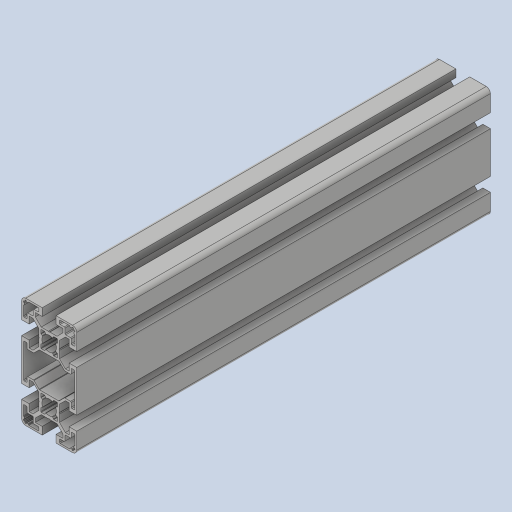
# Autodesk Inventor part: HFSLB8-4080-300
Saved by Autodesk Inventor 2023 (Build 270158000, 158)
## iProperties
Created: 2024-09-13
Part Number: HFSLB8-4080-300
Material: Generic
Catalog Web Link: www.cadenas.de
Description: NEFS8-4080, NEFSB8-4080, NEFSY8-4080, EFS8-4080, EFSB8-4080, HFS8-4080, HFSB8-4080, CAF8-4080, NFSL8-4080, HFSL8-4080, HFSLB8-4080, GFS8-4080, HFSY8-4080-Aluminum Frames -8 Series-2 Row Groove 40x80 mm Square-Specified Length
Vendor: MISUMI
Document SubType Name: Modeling
Designer: psAdmin
Manufacturer: MISUMI
Mass: 238.133 g
Surface Area: 2732.8 cm^2
Volume: 238.133 cm^3
Density: 1 g/cm^3
Appearance: PSOLRGB-175-175-175
Category: PARTsolutions
Company: MISUMI
PSOL_IDENT_0: {$CADENAS_DATA/23d-libs/misumi/metric/38_al_extrusions_blackets/8/hfs8_4080.prj},740 {VTYP=3D},{NB=H
PSOL_IDENT_1: FSLB8-4080-300},{LINA=HFSLB8-4080-300},{NN=NEFS8-4080, NEFSB8-4080, NEFSY8-4080, EFS8-4080, EFSB8-40
PSOL_IDENT_2: 80, HFS8-4080, HFSB8-4080, CAF8-4080, NFSL8-4080, HFSL8-4080, HFSLB8-4080, GFS8-4080, HFSY8-4080},{D
PSOL_IDENT_3: ATE=31.01.2024 10:05:59},{GEOMDATE=26.07.2023 02:49:00},{VERSION=},{LINEID=70},{WBVAR=L,ALT1,ALT2,AL
PSOL_IDENT_4: T4,ALT5,CP5,DL5,DR5,ALT6,ALT9,ALT10,ALT11,HP6,NHL6,DL6,NHR6,DR6,ALT7,ALT8,NH9,AH,BH,CH,DH,EH,NH10,AV
PSOL_IDENT_5: ,BV,CV,DV,EV,NH11,AP,BP,CP,DP,EP,ALT12,ALT13,Z,NH12,XA,XB,XC,XD,XE,NH13,YA,YB,YC,YD,YE,ALT14,HP14,DL
PSOL_IDENT_6: 14,DR14,ALT15,HP15,DL15,DR15,ALT16,HP16,DL16,DR16,ALT17,HQ17,JLP,ALT18,HQ18,KLP,ALT19,ALT20},{WBNUME
PSOL_IDENT_7: RIC=L,NH9,AH,BH,CH,DH,EH,NH10,AV,BV,CV,DV,EV,NH11,AP,BP,CP,DP,EP,NH12,XA,XB,XC,XD,XE,NH13,YA,YB,YC,Y
PSOL_IDENT_8: D,YE,HQ17,JLP,HQ18,KLP}  {NB=HFSLB8-4080-300},{LINA=HFSLB8-4080-300},{KT=DUMMY},{PN=HFSLB8-4080-300}
PSOL_IDENT_9: ,{TPS=HFSLB8-4080},{MAT=A6N01SS-T5 Aluminum Alloy},{ST=Black Anodize},{FRMW=40},{FRMH=80},{FRD=10.5}
PSOL_IDENT_10: ,{L=300},{MASS=2.12},{SA=785},{LX=13.4x10^4},{LY=52.9x10^4},{ALT1=},{M1=0},{IDM1=10.106},{DPL1=0},{D
PSOL_IDENT_11: PR1=0},{ALT1PN=},{ALT2=},{ALT2ALG= '','w/o End Tapping (Insert)','LHP','with LHP (Tapping on the Lef
PSOL_IDENT_12: t (Insert))','RHP','with RHP (Tapping on the Right (Insert))','HPW','with HPW (Tapping on Both Ends
PSOL_IDENT_13: (Insert))' },{M2=0},{DP2=0},{ALT2PN=},{ALT4=},{ALT4ALG= '', 'w/o SC (High Precision Cut)', 'SC', 'wi
PSOL_IDENT_14: th SC (High Precision Cut)' },{ALT4PN=},{ALT5=},{ALT5ALG= '','w/o 45 Degree Cut','1','with 45 Degree
PSOL_IDENT_15: Cut' },{CP5=},{CP5ALG= '','N/A' },{DL5=},{DL5ALG= '','N/A' },{DR5=},{DR5ALG= '','N/A' },{FRMLALT5=0
PSOL_IDENT_16: },{FRMRALT5=0},{ALT5PN=},{ALT6=},{ALT6ALG= '','w/o Fastening Location Wrench Access Hole Alterations'
PSOL_IDENT_17: ,'1','with Fastening Location Wrench Access Hole Alterations' },{ALT9=},{ALT9ALG= '','w/o Location S
PSOL_IDENT_18: pecified Wrench Access Hole Alteratons (Horizontal)','1','with Location Specified Wrench Access Hole
PSOL_IDENT_19: Alteratons (Horizontal)' },{ALT10=},{ALT10ALG= '','w/o Location Specified Wrench Access Hole Altera
PSOL_IDENT_20: tons (Vertical)','1','with Location Specified Wrench Access Hole Alteratons (Vertical)' },{ALT11=},{
PSOL_IDENT_21: ALT11ALG= '','w/o Location Specified Wrench Access Hole Alteratons (Crisscross)','1','with Location
PSOL_IDENT_22: Specified Wrench Access Hole Alteratons (Crisscross)' },{HP6=},{HP6ALG= '','N/A' },{NHL6=},{NHL6ALG=
PSOL_IDENT_23: '','N/A' },{DL6=},{DL6ALG= '','N/A' },{NHR6=},{NHR6ALG= '','N/A' },{DR6=},{DR6ALG= '','N/A' },{HL6=
PSOL_IDENT_24: 0},{HL6D=0},{HR6=0},{HR6D=0},{J6=0},{J6D=0},{K6=0},{K6D=0},{DD6=0},{DD6ALG=0},{ALT7=},{ALT7ALG= '','
PSOL_IDENT_25: N/A' },{ALT8=},{ALT8ALG= '','N/A' },{ALT678PN=},{NH9=0},{NH9MAX=5},{NH9ALG=[0]},{AH=0.0},{AHMIN=7},{
PSOL_IDENT_26: AHMAX=295},{AHALG=[0]},{BH=0.0},{BHMIN=2},{BHMAX=297},{BHALG=[0]},{CH=0.0},{CHMIN=2},{CHMAX=299},{CH
PSOL_IDENT_27: ALG=[0]},{DH=0.0},{DHMIN=2},{DHMAX=301},{DHALG=[0]},{EH=0.0},{EHMIN=2},{EHMAX=293},{EHALG=[0]},{NH10=
PSOL_IDENT_28: 0},{NH10MAX=5},{NH10ALG=[0]},{AV=0.0},{AVMIN=7},{AVMAX=295},{AVALG=[0]},{BV=0.0},{BVMIN=2},{BVMAX=29
PSOL_IDENT_29: 7},{BVALG=[0]},{CV=0.0},{CVMIN=2},{CVMAX=299},{CVALG=[0]},{DV=0.0},{DVMIN=2},{DVMAX=301},{DVALG=[0]}
PSOL_IDENT_30: ,{EV=0.0},{EVMIN=2},{EVMAX=293},{EVALG=[0]},{NH11=0},{NH11MAX=5},{NH11ALG=[0]},{AP=0.0},{APMIN=7},{A
PSOL_IDENT_31: PMAX=295},{APALG=[0]},{BP=0.0},{BPMIN=2},{BPMAX=297},{BPALG=[0]},{CP=0.0},{CPMIN=2},{CPMAX=299},{CPA
PSOL_IDENT_32: LG=[0]},{DP=0.0},{DPMIN=2},{DPMAX=301},{DPALG=[0]},{EP=0.0},{EPMIN=2},{EPMAX=293},{EPALG=[0]},{ALT9P
PSOL_IDENT_33: N=},{ALT10PN=},{ALT11PN=},{ALT91011PN=},{ALT12=},{ALT12ALG= '','w/o Counterbore Hole in Specified Po
PSOL_IDENT_34: sition (Vertical)','1','with Counterbore Hole in Specified Position (Vertical)' },{ALT13=},{ALT13ALG=
PSOL_IDENT_35: '','w/o Counterbore Hole in Specified Position (Horizontal)','1','with Counterbore Hole in Specifie
PSOL_IDENT_36: d Position (Horizontal)' },{Z=},{ZALG= '','N/A' },{DD12=0.0},{DD112=0.0},{NH12=0},{NH12MAX=5},{NH12A
PSOL_IDENT_37: LG=[0]},{XA=0.0},{XAMIN=7},{XAMAX=295},{XAALG=[0]},{XB=0.0},{XBMIN=2},{XBMAX=297},{XBALG=[0]},{XC=0.
PSOL_IDENT_38: 0},{XCMIN=2},{XCMAX=299},{XCALG=[0]},{XD=0.0},{XDMIN=2},{XDMAX=301},{XDALG=[0]},{XE=0.0},{XEMIN=2},{
PSOL_IDENT_39: XEMAX=293},{XEALG=[0]},{NH13=0},{NH13MAX=5},{NH13ALG=[0]},{YA=0.0},{YAMIN=7},{YAMAX=295},{YAALG=[0]}
PSOL_IDENT_40: ,{YB=0.0},{YBMIN=2},{YBMAX=297},{YBALG=[0]},{YC=0.0},{YCMIN=2},{YCMAX=299},{YCALG=[0]},{YD=0.0},{YDM
PSOL_IDENT_41: IN=2},{YDMAX=301},{YDALG=[0]},{YE=0.0},{YEMIN=2},{YEMAX=293},{YEALG=[0]},{ALT12PN=},{ALT13PN=},{ALT1
PSOL_IDENT_42: 213PN=},{ALT14=},{ALT14ALG= '','w/o D Type Hole Alteration','1','with D Type Hole Alteration' },{HP1
PSOL_IDENT_43: 4=},{HP14ALG= '','N/A' },{DL14=},{DL14ALG= '','N/A' },{DR14=},{DR14ALG= '','N/A' },{H14=0},{D14=0.0}
PSOL_IDENT_44: ,{ALT14PN=},{ALT15=},{ALT15ALG= '','w/o S Type Hole Alteration','1','with S Type Hole Alteration' },
PSOL_IDENT_45: {HP15=},{HP15ALG= '','N/A' },{DL15=},{DL15ALG= '','N/A' },{DR15=},{DR15ALG= '','N/A' },{H15=0},{D115=
PSOL_IDENT_46: 0.0},{D215=0.0},{ALT15PN=},{ALT16=},{ALT16ALG= '','w/o M Type Hole Alteration','1','with M Type Hole
PSOL_IDENT_47: Alteration' },{HP16=},{HP16ALG= '','N/A' },{DL16=},{DL16ALG= '','N/A' },{DR16=},{DR16ALG= '','N/A'
PSOL_IDENT_48: },{H116=0},{D16=0.0},{ALT16PN=},{ALT17=},{ALT17ALG= '','w/o L Type Hole Alteration (Top)','1','with
PSOL_IDENT_49: L Type Hole Alteration (Top)' },{HQ17=0},{HQ17ALG=0},{JLP=0},{JLPMIN=4.9},{JLPMAX=0},{JLPALG=[0]},{L
PSOL_IDENT_50: 17=0},{D17=0.0},{ALT18=},{ALT18ALG= '','w/o L Type Hole Alteration (Bottom)','1','with L Type Hole A
PSOL_IDENT_51: lteration (Bottom)' },{HQ18=0},{HQ18ALG=0},{KLP=0},{KLPMIN=4.9},{KLPMAX=0},{KLPALG=[0]},{L18=0},{D18=
PSOL_IDENT_52: 0.0},{ALT1718PN=},{ALT19=},{ALT19ALG= '','N/A' },{M19=0},{DP19=0},{ALT19PN=},{ALT20=},{ALT20PN=},{ER
PSOL_IDENT_53: RORALT01=OK},{ERRORALT02=OK},{ERRORALT05=OK},{ERRORALT06091=OK},{ERRORALT06092=OK},{ERRORALT06093=OK
PSOL_IDENT_54: },{ERRORALT06094=OK},{ERRORALT06101=OK},{ERRORALT06102=OK},{ERRORALT06103=OK},{ERRORALT06104=OK},{ER
PSOL_IDENT_55: RORALT06111=OK},{ERRORALT06112=OK},{ERRORALT06113=OK},{ERRORALT06114=OK},{ERRORALT06121=OK},{ERRORAL
PSOL_IDENT_56: T06122=OK},{ERRORALT06123=OK},{ERRORALT06124=OK},{ERRORALT06131=OK},{ERRORALT06132=OK},{ERRORALT0613
PSOL_IDENT_57: 3=OK},{ERRORALT06134=OK},{ERRORALT0614=OK},{ERRORALT0615=OK},{ERRORALT0616=OK},{ERRORALT06171=OK},{E
PSOL_IDENT_58: RRORALT06172=OK},{ERRORALT06173=OK},{ERRORALT06181=OK},{ERRORALT06182=OK},{ERRORALT06183=OK},{ERRORA
PSOL_IDENT_59: LT0619=OK},{ERRORALT0911=OK},{ERRORALT0913=OK},{ERRORALT0914=OK},{ERRORALT0915=OK},{ERRORALT0916=OK}
PSOL_IDENT_60: ,{ERRORALT0917=OK},{ERRORALT0918=OK},{ERRORALT0919=OK},{ERRORALT1011=OK},{ERRORALT1012=OK},{ERRORALT
PSOL_IDENT_61: 1014=OK},{ERRORALT1015=OK},{ERRORALT1016=OK},{ERRORALT1017=OK},{ERRORALT1018=OK},{ERRORALT1019=OK},{
PSOL_IDENT_62: ERRORALT1112=OK},{ERRORALT1113=OK},{ERRORALT1114=OK},{ERRORALT1115=OK},{ERRORALT1116=OK},{ERRORALT11
PSOL_IDENT_63: 17=OK},{ERRORALT1118=OK},{ERRORALT1119=OK},{ERRORALT1214=OK},{ERRORALT1215=OK},{ERRORALT1216=OK},{ER
PSOL_IDENT_64: RORALT1217=OK},{ERRORALT1218=OK},{ERRORALT1219=OK},{ERRORALT1314=OK},{ERRORALT1315=OK},{ERRORALT1316=
PSOL_IDENT_65: OK},{ERRORALT1317=OK},{ERRORALT1318=OK},{ERRORALT1319=OK},{ERRORALT1415=OK},{ERRORALT1416=OK},{ERROR
PSOL_IDENT_66: ALT1417=OK},{ERRORALT1418=OK},{ERRORALT1419=OK},{ERRORALT1516=OK},{ERRORALT1517=OK},{ERRORALT1518=OK
PSOL_IDENT_67: },{ERRORALT1519=OK},{ERRORALT1617=OK},{ERRORALT1618=OK},{ERRORALT1619=OK},{ERRORALT1719=OK},{ERRORAL
PSOL_IDENT_68: T1819=OK},{ERRORPN=},{COLOR=}
NB: HFSLB8-4080-300
NN: NEFS8-4080, NEFSB8-4080, NEFSY8-4080, EFS8-4080, EFSB8-4080, HFS8-4080, HFSB8-4080, CAF8-4080, NFSL8-4080, HFSL8-4080, HFSLB8-4080, GFS8-4080, HFSY8-4080
NT: Aluminum Frames -8 Series-2 Row Groove 40x80 mm Square-Specified Length
NBSYN: $PN.
LINA: HFSLB8-4080-300
CATALOG: Misumi
PN: HFSLB8-4080-300
TPS: HFSLB8-4080
MAT: A6N01SS-T5 Aluminum Alloy
ST: Black Anodize
L: 300
MASS: 2.12
SA: 785
LX: 13.4x10^4
LY: 52.9x10^4
ALT1: w/o End Tapping
M1: 0
DPL1: 0
DPR1: 0
ALT2: w/o End Tapping (Insert)
M2: 0
DP2: 0
ALT4: w/o SC (High Precision Cut)
ALT5: w/o 45 Degree Cut
CP5: N/A
DL5: N/A
DR5: N/A
ALT6: w/o Fastening Location Wrench Access Hole Alterations
ALT9: w/o Location Specified Wrench Access Hole Alteratons (Horizontal)
ALT10: w/o Location Specified Wrench Access Hole Alteratons (Vertical)
ALT11: w/o Location Specified Wrench Access Hole Alteratons (Crisscross)
HP6: N/A
NHL6: N/A
DL6: N/A
NHR6: N/A
DR6: N/A
HL6D: 0
HR6D: 0
J6D: 0
K6D: 0
DD6: 0
ALT7: N/A
ALT8: N/A
NH9: 0
AH: 0
BH: 0
CH: 0
DH: 0
EH: 0
NH10: 0
AV: 0
BV: 0
CV: 0
DV: 0
EV: 0
NH11: 0
AP: 0
BP: 0
CP: 0
DP: 0
EP: 0
ALT12: w/o Counterbore Hole in Specified Position (Vertical)
ALT13: w/o Counterbore Hole in Specified Position (Horizontal)
Z: N/A
DD12: 0
DD112: 0
NH12: 0
XA: 0
XB: 0
XC: 0
XD: 0
XE: 0
NH13: 0
YA: 0
YB: 0
YC: 0
YD: 0
YE: 0
ALT14: w/o D Type Hole Alteration
HP14: N/A
DL14: N/A
DR14: N/A
H14: 0
D14: 0
ALT15: w/o S Type Hole Alteration
HP15: N/A
DL15: N/A
DR15: N/A
H15: 0
D115: 0
D215: 0
ALT16: w/o M Type Hole Alteration
HP16: N/A
DL16: N/A
DR16: N/A
H116: 0
D16: 0
ALT17: w/o L Type Hole Alteration (Top)
HQ17: 0
JLP: 0
D17: 0
ALT18: w/o L Type Hole Alteration (Bottom)
HQ18: 0
KLP: 0
D18: 0
ALT19: N/A
M19: 0
DP19: 0
ALT20: w/o CW (End Face C Chamfering)
SUPPLIER: MISUMI
ARTICLENO: HFSLB8-4080-300
BOMINFO: HFSLB8-4080-300
CREATOR: CADENAS GmbH
Title: HFSLB8-4080-300
Author: Cadenas PARTsolutions
Comments: Aluminum Frames -8 Series-2 Row Groove 40x80 mm Square-Specified Length
Autodesk Inventor part; units mm, degrees
sketch "Sketch_59" plane through (0, 0, 0) normal (0, 0, 1) x (1, 0, 0)
  arc A0 (-20, -37) -> (-17, -40) centre (-17, -37) ccw
  line L0 (-17, -40) -> (-5, -40)
  line L1 (-5, -40) -> (-5, -34.5)
  line L2 (-5, -34.5) -> (-10, -34.5)
  line L3 (-10, -34.5) -> (-10, -31.7678)
  line L4 (-10, -31.7678) -> (-5.7322, -27.5)
  line L5 (-5.7322, -27.5) -> (-0.5196, -27.5)
  line L6 (-0.5196, -27.5) -> (0, -27.2)
  line L7 (0, -27.2) -> (0.5196, -27.5)
  line L8 (0.5196, -27.5) -> (5.7322, -27.5)
  line L9 (5.7322, -27.5) -> (10, -31.7678)
  line L10 (10, -31.7678) -> (10, -34.5)
  line L11 (10, -34.5) -> (5, -34.5)
  line L12 (5, -34.5) -> (5, -40)
  line L13 (5, -40) -> (17, -40)
  arc A1 (17, -40) -> (20, -37) centre (17, -37) ccw
  line L14 (20, -37) -> (20, -25)
  line L15 (20, -25) -> (14.5, -25)
  line L16 (14.5, -25) -> (14.5, -30)
  line L17 (14.5, -30) -> (11.7678, -30)
  line L18 (11.7678, -30) -> (7.5, -25.7322)
  line L19 (7.5, -25.7322) -> (7.5, -20.5196)
  line L20 (7.5, -20.5196) -> (7.2, -20)
  line L21 (7.2, -20) -> (7.5, -19.4804)
  line L22 (7.5, -19.4804) -> (7.5, -14.2678)
  line L23 (7.5, -14.2678) -> (11.7678, -10)
  line L24 (11.7678, -10) -> (14.5, -10)
  line L25 (14.5, -10) -> (14.5, -15)
  line L26 (14.5, -15) -> (20, -15)
  line L27 (20, -15) -> (20, 15)
  line L28 (20, 15) -> (14.5, 15)
  line L29 (14.5, 15) -> (14.5, 10)
  line L30 (14.5, 10) -> (11.7678, 10)
  line L31 (11.7678, 10) -> (7.5, 14.2678)
  line L32 (7.5, 14.2678) -> (7.5, 19.4804)
  line L33 (7.5, 19.4804) -> (7.2, 20)
  line L34 (7.2, 20) -> (7.5, 20.5196)
  line L35 (7.5, 20.5196) -> (7.5, 25.7322)
  line L36 (7.5, 25.7322) -> (11.7678, 30)
  line L37 (11.7678, 30) -> (14.5, 30)
  line L38 (14.5, 30) -> (14.5, 25)
  line L39 (14.5, 25) -> (20, 25)
  line L40 (20, 25) -> (20, 37)
  arc A2 (20, 37) -> (17, 40) centre (17, 37) ccw
  line L41 (17, 40) -> (5, 40)
  line L42 (5, 40) -> (5, 34.5)
  line L43 (5, 34.5) -> (10, 34.5)
  line L44 (10, 34.5) -> (10, 31.7678)
  line L45 (10, 31.7678) -> (5.7322, 27.5)
  line L46 (5.7322, 27.5) -> (0.5196, 27.5)
  line L47 (0.5196, 27.5) -> (0, 27.2)
  line L48 (0, 27.2) -> (-0.5196, 27.5)
  line L49 (-0.5196, 27.5) -> (-5.7322, 27.5)
  line L50 (-5.7322, 27.5) -> (-10, 31.7678)
  line L51 (-10, 31.7678) -> (-10, 34.5)
  line L52 (-10, 34.5) -> (-5, 34.5)
  line L53 (-5, 34.5) -> (-5, 40)
  line L54 (-5, 40) -> (-17, 40)
  arc A3 (-17, 40) -> (-20, 37) centre (-17, 37) ccw
  line L55 (-20, 37) -> (-20, 25)
  line L56 (-20, 25) -> (-14.5, 25)
  line L57 (-14.5, 25) -> (-14.5, 30)
  line L58 (-14.5, 30) -> (-11.7678, 30)
  line L59 (-11.7678, 30) -> (-7.5, 25.7322)
  line L60 (-7.5, 25.7322) -> (-7.5, 20.5196)
  line L61 (-7.5, 20.5196) -> (-7.2, 20)
  line L62 (-7.2, 20) -> (-7.5, 19.4804)
  line L63 (-7.5, 19.4804) -> (-7.5, 14.2678)
  line L64 (-7.5, 14.2678) -> (-11.7678, 10)
  line L65 (-11.7678, 10) -> (-14.5, 10)
  line L66 (-14.5, 10) -> (-14.5, 15)
  line L67 (-14.5, 15) -> (-20, 15)
  line L68 (-20, 15) -> (-20, -15)
  line L69 (-20, -15) -> (-14.5, -15)
  line L70 (-14.5, -15) -> (-14.5, -10)
  line L71 (-14.5, -10) -> (-11.7678, -10)
  line L72 (-11.7678, -10) -> (-7.5, -14.2678)
  line L73 (-7.5, -14.2678) -> (-7.5, -19.4804)
  line L74 (-7.5, -19.4804) -> (-7.2, -20)
  line L75 (-7.2, -20) -> (-7.5, -20.5196)
  line L76 (-7.5, -20.5196) -> (-7.5, -25.7322)
  line L77 (-7.5, -25.7322) -> (-11.7678, -30)
  line L78 (-11.7678, -30) -> (-14.5, -30)
  line L79 (-14.5, -30) -> (-14.5, -25)
  line L80 (-14.5, -25) -> (-20, -25)
  line L81 (-20, -25) -> (-20, -37)
  line L82 (7.5, -36.5) -> (7.5, -38.2)
  arc A4 (7.5, -38.2) -> (8, -38.7) centre (8, -38.2) ccw
  line L83 (8, -38.7) -> (14.7, -38.7)
  arc A5 (14.7, -38.7) -> (15, -38.4) centre (14.7, -38.4) ccw
  line L84 (15, -38.4) -> (15, -38.3)
  arc A6 (15.3, -38) -> (15, -38.3) centre (15.3, -38.3) ccw
  line L85 (15.3, -38) -> (16.3, -38)
  arc A7 (16.6, -38.3) -> (16.3, -38) centre (16.3, -38.3) ccw
  line L86 (16.6, -38.3) -> (16.6, -38.4)
  arc A8 (16.6, -38.4) -> (16.9, -38.7) centre (16.9, -38.4) ccw
  line L87 (16.9, -38.7) -> (17.3, -38.7)
  arc A9 (17.3, -38.7) -> (17.6, -38.4) centre (17.3, -38.4) ccw
  line L88 (17.6, -38.4) -> (17.6, -37.9)
  arc A10 (17.9, -37.6) -> (17.6, -37.9) centre (17.9, -37.9) ccw
  line L89 (17.9, -37.6) -> (18.4, -37.6)
  arc A11 (18.4, -37.6) -> (18.7, -37.3) centre (18.4, -37.3) ccw
  line L90 (18.7, -37.3) -> (18.7, -36.9)
  arc A12 (18.7, -36.9) -> (18.4, -36.6) centre (18.4, -36.9) ccw
  line L91 (18.4, -36.6) -> (18.3, -36.6)
  arc A13 (18, -36.3) -> (18.3, -36.6) centre (18.3, -36.3) ccw
  line L92 (18, -36.3) -> (18, -35.3)
  arc A14 (18.3, -35) -> (18, -35.3) centre (18.3, -35.3) ccw
  line L93 (18.3, -35) -> (18.4, -35)
  arc A15 (18.4, -35) -> (18.7, -34.7) centre (18.4, -34.7) ccw
  line L94 (18.7, -34.7) -> (18.7, -28)
  arc A16 (18.7, -28) -> (18.2, -27.5) centre (18.2, -28) ccw
  line L95 (18.2, -27.5) -> (16.5, -27.5)
  arc A17 (16.5, -27.5) -> (16, -28) centre (16.5, -28) ccw
  line L96 (16, -28) -> (16, -31)
  arc A18 (15.5, -31.5) -> (16, -31) centre (15.5, -31) ccw
  line L97 (15.5, -31.5) -> (12, -31.5)
  arc A19 (12, -31.5) -> (11.5, -32) centre (12, -32) ccw
  line L98 (11.5, -32) -> (11.5, -35.5)
  arc A20 (11, -36) -> (11.5, -35.5) centre (11, -35.5) ccw
  line L99 (11, -36) -> (8, -36)
  arc A21 (8, -36) -> (7.5, -36.5) centre (8, -36.5) ccw
  line L100 (7.5, 38.2) -> (7.5, 36.5)
  arc A22 (7.5, 36.5) -> (8, 36) centre (8, 36.5) ccw
  line L101 (8, 36) -> (11, 36)
  arc A23 (11.5, 35.5) -> (11, 36) centre (11, 35.5) ccw
  line L102 (11.5, 35.5) -> (11.5, 32)
  arc A24 (11.5, 32) -> (12, 31.5) centre (12, 32) ccw
  line L103 (12, 31.5) -> (15.5, 31.5)
  arc A25 (16, 31) -> (15.5, 31.5) centre (15.5, 31) ccw
  line L104 (16, 31) -> (16, 28)
  arc A26 (16, 28) -> (16.5, 27.5) centre (16.5, 28) ccw
  line L105 (16.5, 27.5) -> (18.2, 27.5)
  arc A27 (18.2, 27.5) -> (18.7, 28) centre (18.2, 28) ccw
  line L106 (18.7, 28) -> (18.7, 34.7)
  arc A28 (18.7, 34.7) -> (18.4, 35) centre (18.4, 34.7) ccw
  line L107 (18.4, 35) -> (18.3, 35)
  arc A29 (18, 35.3) -> (18.3, 35) centre (18.3, 35.3) ccw
  line L108 (18, 35.3) -> (18, 36.3)
  arc A30 (18.3, 36.6) -> (18, 36.3) centre (18.3, 36.3) ccw
  line L109 (18.3, 36.6) -> (18.4, 36.6)
  arc A31 (18.4, 36.6) -> (18.7, 36.9) centre (18.4, 36.9) ccw
  line L110 (18.7, 36.9) -> (18.7, 37.3)
  arc A32 (18.7, 37.3) -> (18.4, 37.6) centre (18.4, 37.3) ccw
  line L111 (18.4, 37.6) -> (17.9, 37.6)
  arc A33 (17.6, 37.9) -> (17.9, 37.6) centre (17.9, 37.9) ccw
  line L112 (17.6, 37.9) -> (17.6, 38.4)
  arc A34 (17.6, 38.4) -> (17.3, 38.7) centre (17.3, 38.4) ccw
  line L113 (17.3, 38.7) -> (16.9, 38.7)
  arc A35 (16.9, 38.7) -> (16.6, 38.4) centre (16.9, 38.4) ccw
  line L114 (16.6, 38.4) -> (16.6, 38.3)
  arc A36 (16.3, 38) -> (16.6, 38.3) centre (16.3, 38.3) ccw
  line L115 (16.3, 38) -> (15.3, 38)
  arc A37 (15, 38.3) -> (15.3, 38) centre (15.3, 38.3) ccw
  line L116 (15, 38.3) -> (15, 38.4)
  arc A38 (15, 38.4) -> (14.7, 38.7) centre (14.7, 38.4) ccw
  line L117 (14.7, 38.7) -> (8, 38.7)
  arc A39 (8, 38.7) -> (7.5, 38.2) centre (8, 38.2) ccw
  line L118 (-18.5, 12) -> (-18.5, -12)
  arc A40 (-18.5, -12) -> (-18, -12.5) centre (-18, -12) ccw
  line L119 (-18, -12.5) -> (-16.5, -12.5)
  arc A41 (-16.5, -12.5) -> (-16, -12) centre (-16.5, -12) ccw
  line L120 (-16, -12) -> (-16, -9)
  arc A42 (-15.5, -8.5) -> (-16, -9) centre (-15.5, -9) ccw
  line L121 (-15.5, -8.5) -> (-11.3536, -8.5)
  arc A43 (-11, -8.6464) -> (-11.3536, -8.5) centre (-11.3536, -9) ccw
  line L122 (-11, -8.6464) -> (-7.2929, -12.3536)
  arc A44 (-7.2929, -12.3536) -> (-6.9393, -12.5) centre (-6.9393, -12) ccw
  line L123 (-6.9393, -12.5) -> (6.9393, -12.5)
  arc A45 (6.9393, -12.5) -> (7.2929, -12.3536) centre (6.9393, -12) ccw
  line L124 (7.2929, -12.3536) -> (11, -8.6464)
  arc A46 (11.3536, -8.5) -> (11, -8.6464) centre (11.3536, -9) ccw
  line L125 (11.3536, -8.5) -> (15.5, -8.5)
  arc A47 (16, -9) -> (15.5, -8.5) centre (15.5, -9) ccw
  line L126 (16, -9) -> (16, -12)
  arc A48 (16, -12) -> (16.5, -12.5) centre (16.5, -12) ccw
  line L127 (16.5, -12.5) -> (18, -12.5)
  arc A49 (18, -12.5) -> (18.5, -12) centre (18, -12) ccw
  line L128 (18.5, -12) -> (18.5, 12)
  arc A50 (18.5, 12) -> (18, 12.5) centre (18, 12) ccw
  line L129 (18, 12.5) -> (16.5, 12.5)
  arc A51 (16.5, 12.5) -> (16, 12) centre (16.5, 12) ccw
  line L130 (16, 12) -> (16, 9)
  arc A52 (15.5, 8.5) -> (16, 9) centre (15.5, 9) ccw
  line L131 (15.5, 8.5) -> (11.3536, 8.5)
  arc A53 (11, 8.6464) -> (11.3536, 8.5) centre (11.3536, 9) ccw
  line L132 (11, 8.6464) -> (7.2929, 12.3536)
  arc A54 (7.2929, 12.3536) -> (6.9393, 12.5) centre (6.9393, 12) ccw
  line L133 (6.9393, 12.5) -> (-6.9393, 12.5)
  arc A55 (-6.9393, 12.5) -> (-7.2929, 12.3536) centre (-6.9393, 12) ccw
  line L134 (-7.2929, 12.3536) -> (-11, 8.6464)
  arc A56 (-11.3536, 8.5) -> (-11, 8.6464) centre (-11.3536, 9) ccw
  line L135 (-11.3536, 8.5) -> (-15.5, 8.5)
  arc A57 (-16, 9) -> (-15.5, 8.5) centre (-15.5, 9) ccw
  line L136 (-16, 9) -> (-16, 12)
  arc A58 (-16, 12) -> (-16.5, 12.5) centre (-16.5, 12) ccw
  line L137 (-16.5, 12.5) -> (-18, 12.5)
  arc A59 (-18, 12.5) -> (-18.5, 12) centre (-18, 12) ccw
  line L138 (-18.7, 37.3) -> (-18.7, 36.9)
  arc A60 (-18.7, 36.9) -> (-18.4, 36.6) centre (-18.4, 36.9) ccw
  line L139 (-18.4, 36.6) -> (-18.3, 36.6)
  arc A61 (-18, 36.3) -> (-18.3, 36.6) centre (-18.3, 36.3) ccw
  line L140 (-18, 36.3) -> (-18, 35.3)
  arc A62 (-18.3, 35) -> (-18, 35.3) centre (-18.3, 35.3) ccw
  line L141 (-18.3, 35) -> (-18.4, 35)
  arc A63 (-18.4, 35) -> (-18.7, 34.7) centre (-18.4, 34.7) ccw
  line L142 (-18.7, 34.7) -> (-18.7, 28)
  arc A64 (-18.7, 28) -> (-18.2, 27.5) centre (-18.2, 28) ccw
  line L143 (-18.2, 27.5) -> (-16.5, 27.5)
  arc A65 (-16.5, 27.5) -> (-16, 28) centre (-16.5, 28) ccw
  line L144 (-16, 28) -> (-16, 31)
  arc A66 (-15.5, 31.5) -> (-16, 31) centre (-15.5, 31) ccw
  line L145 (-15.5, 31.5) -> (-12, 31.5)
  arc A67 (-12, 31.5) -> (-11.5, 32) centre (-12, 32) ccw
  line L146 (-11.5, 32) -> (-11.5, 35.5)
  arc A68 (-11, 36) -> (-11.5, 35.5) centre (-11, 35.5) ccw
  line L147 (-11, 36) -> (-8, 36)
  arc A69 (-8, 36) -> (-7.5, 36.5) centre (-8, 36.5) ccw
  line L148 (-7.5, 36.5) -> (-7.5, 38.2)
  arc A70 (-7.5, 38.2) -> (-8, 38.7) centre (-8, 38.2) ccw
  line L149 (-8, 38.7) -> (-14.7, 38.7)
  arc A71 (-14.7, 38.7) -> (-15, 38.4) centre (-14.7, 38.4) ccw
  line L150 (-15, 38.4) -> (-15, 38.3)
  arc A72 (-15.3, 38) -> (-15, 38.3) centre (-15.3, 38.3) ccw
  line L151 (-15.3, 38) -> (-16.3, 38)
  arc A73 (-16.6, 38.3) -> (-16.3, 38) centre (-16.3, 38.3) ccw
  line L152 (-16.6, 38.3) -> (-16.6, 38.4)
  arc A74 (-16.6, 38.4) -> (-16.9, 38.7) centre (-16.9, 38.4) ccw
  line L153 (-16.9, 38.7) -> (-17.3, 38.7)
  arc A75 (-17.3, 38.7) -> (-17.6, 38.4) centre (-17.3, 38.4) ccw
  line L154 (-17.6, 38.4) -> (-17.6, 37.9)
  arc A76 (-17.9, 37.6) -> (-17.6, 37.9) centre (-17.9, 37.9) ccw
  line L155 (-17.9, 37.6) -> (-18.4, 37.6)
  arc A77 (-18.4, 37.6) -> (-18.7, 37.3) centre (-18.4, 37.3) ccw
  arc A78 (-18.7, -37.3) -> (-18.4, -37.6) centre (-18.4, -37.3) ccw
  line L156 (-18.4, -37.6) -> (-17.9, -37.6)
  arc A79 (-17.6, -37.9) -> (-17.9, -37.6) centre (-17.9, -37.9) ccw
  line L157 (-17.6, -37.9) -> (-17.6, -38.4)
  arc A80 (-17.6, -38.4) -> (-17.3, -38.7) centre (-17.3, -38.4) ccw
  line L158 (-17.3, -38.7) -> (-16.9, -38.7)
  arc A81 (-16.9, -38.7) -> (-16.6, -38.4) centre (-16.9, -38.4) ccw
  line L159 (-16.6, -38.4) -> (-16.6, -38.3)
  arc A82 (-16.3, -38) -> (-16.6, -38.3) centre (-16.3, -38.3) ccw
  line L160 (-16.3, -38) -> (-15.3, -38)
  arc A83 (-15, -38.3) -> (-15.3, -38) centre (-15.3, -38.3) ccw
  line L161 (-15, -38.3) -> (-15, -38.4)
  arc A84 (-15, -38.4) -> (-14.7, -38.7) centre (-14.7, -38.4) ccw
  line L162 (-14.7, -38.7) -> (-8, -38.7)
  arc A85 (-8, -38.7) -> (-7.5, -38.2) centre (-8, -38.2) ccw
  line L163 (-7.5, -38.2) -> (-7.5, -36.5)
  arc A86 (-7.5, -36.5) -> (-8, -36) centre (-8, -36.5) ccw
  line L164 (-8, -36) -> (-11, -36)
  arc A87 (-11.5, -35.5) -> (-11, -36) centre (-11, -35.5) ccw
  line L165 (-11.5, -35.5) -> (-11.5, -32)
  arc A88 (-11.5, -32) -> (-12, -31.5) centre (-12, -32) ccw
  line L166 (-12, -31.5) -> (-15.5, -31.5)
  arc A89 (-16, -31) -> (-15.5, -31.5) centre (-15.5, -31) ccw
  line L167 (-16, -31) -> (-16, -28)
  arc A90 (-16, -28) -> (-16.5, -27.5) centre (-16.5, -28) ccw
  line L168 (-16.5, -27.5) -> (-18.2, -27.5)
  arc A91 (-18.2, -27.5) -> (-18.7, -28) centre (-18.2, -28) ccw
  line L169 (-18.7, -28) -> (-18.7, -34.7)
  arc A92 (-18.7, -34.7) -> (-18.4, -35) centre (-18.4, -34.7) ccw
  line L170 (-18.4, -35) -> (-18.3, -35)
  arc A93 (-18, -35.3) -> (-18.3, -35) centre (-18.3, -35.3) ccw
  line L171 (-18, -35.3) -> (-18, -36.3)
  arc A94 (-18.3, -36.6) -> (-18, -36.3) centre (-18.3, -36.3) ccw
  line L172 (-18.3, -36.6) -> (-18.4, -36.6)
  arc A95 (-18.4, -36.6) -> (-18.7, -36.9) centre (-18.4, -36.9) ccw
  line L173 (-18.7, -36.9) -> (-18.7, -37.3)
  constraints: 348 end point, 192 point on circle, 96 centre point
extrude "Extrusion1" add sketch "Sketch_59" against normal blind 300
sketch "Sketch_94" plane through (0, 0, 0) normal (0, 0, 1) x (1, 0, 0)
  line L0 (-6, 16.62) -> (-6, 14.3)
  arc A0 (-6, 14.3) -> (-5.7, 14) centre (-5.7, 14.3) ccw
  line L1 (-5.7, 14) -> (-3.38, 14)
  arc A1 (-3.38, 14) -> (-3.1153, 14.1588) centre (-3.38, 14.3) ccw
  line L2 (-3.1153, 14.1588) -> (-2.6079, 15.1101)
  arc A2 (-2.2166, 15.2409) -> (-2.6079, 15.1101) centre (-2.3432, 14.9689) ccw
  arc A3 (-2.2166, 15.2409) -> (2.2166, 15.2409) centre (0, 20) ccw
  arc A4 (2.6079, 15.1101) -> (2.2166, 15.2409) centre (2.3432, 14.9689) ccw
  line L3 (2.6079, 15.1101) -> (3.1153, 14.1588)
  arc A5 (3.1153, 14.1588) -> (3.38, 14) centre (3.38, 14.3) ccw
  line L4 (3.38, 14) -> (5.7, 14)
  arc A6 (5.7, 14) -> (6, 14.3) centre (5.7, 14.3) ccw
  line L5 (6, 14.3) -> (6, 16.62)
  arc A7 (6, 16.62) -> (5.8412, 16.8847) centre (5.7, 16.62) ccw
  line L6 (5.8412, 16.8847) -> (4.8899, 17.3921)
  arc A8 (4.7591, 17.7834) -> (4.8899, 17.3921) centre (5.0311, 17.6568) ccw
  arc A9 (4.7591, 17.7834) -> (4.7591, 22.2166) centre (0, 20) ccw
  arc A10 (4.8899, 22.6079) -> (4.7591, 22.2166) centre (5.0311, 22.3432) ccw
  line L7 (4.8899, 22.6079) -> (5.8412, 23.1153)
  arc A11 (5.8412, 23.1153) -> (6, 23.38) centre (5.7, 23.38) ccw
  line L8 (6, 23.38) -> (6, 25.7)
  arc A12 (6, 25.7) -> (5.7, 26) centre (5.7, 25.7) ccw
  line L9 (5.7, 26) -> (3.38, 26)
  arc A13 (3.38, 26) -> (3.1153, 25.8412) centre (3.38, 25.7) ccw
  line L10 (3.1153, 25.8412) -> (2.6079, 24.8899)
  arc A14 (2.2166, 24.7591) -> (2.6079, 24.8899) centre (2.3432, 25.0311) ccw
  arc A15 (2.2166, 24.7591) -> (-2.2166, 24.7591) centre (0, 20) ccw
  arc A16 (-2.6079, 24.8899) -> (-2.2166, 24.7591) centre (-2.3432, 25.0311) ccw
  line L11 (-2.6079, 24.8899) -> (-3.1153, 25.8412)
  arc A17 (-3.1153, 25.8412) -> (-3.38, 26) centre (-3.38, 25.7) ccw
  line L12 (-3.38, 26) -> (-5.7, 26)
  arc A18 (-5.7, 26) -> (-6, 25.7) centre (-5.7, 25.7) ccw
  line L13 (-6, 25.7) -> (-6, 23.38)
  arc A19 (-6, 23.38) -> (-5.8412, 23.1153) centre (-5.7, 23.38) ccw
  line L14 (-5.8412, 23.1153) -> (-4.8899, 22.6079)
  arc A20 (-4.7591, 22.2166) -> (-4.8899, 22.6079) centre (-5.0311, 22.3432) ccw
  arc A21 (-4.7591, 22.2166) -> (-4.7591, 17.7834) centre (0, 20) ccw
  arc A22 (-4.8899, 17.3921) -> (-4.7591, 17.7834) centre (-5.0311, 17.6568) ccw
  line L15 (-4.8899, 17.3921) -> (-5.8412, 16.8847)
  arc A23 (-5.8412, 16.8847) -> (-6, 16.62) centre (-5.7, 16.62) ccw
  constraints: 48 point on circle, 32 end point, 24 centre point
extrude "Extrusion2" cut sketch "Sketch_94" against normal blind 300
pattern_linear "Rectangular Pattern1" count 2 spacing 40 along (0, -1, 0) of "Extrusion2"
ref_plane "C1_XY" through (0, 0, 0) normal (0, 0, 1) x (1, 0, 0)
ref_plane "C1_YZ" through (0, 0, 0) normal (1, 0, 0) x (0, 1, 0)
ref_plane "C1_ZX" through (0, 0, 0) normal (0, 1, 0) x (0, 0, 1)
ref_plane "to_frame_cap1_XY" through (0, 0, 0) normal (0, 0, 1) x (1, 0, 0)
ref_plane "to_frame_cap1_YZ" through (0, 0, 0) normal (1, 0, 0) x (0, 1, 0)
ref_plane "to_frame_cap1_ZX" through (0, 0, 0) normal (0, 1, 0) x (0, 0, 1)
ref_plane "to_frame_cap2_XY" through (0, 0, -300) normal (0, 0, -1) x (1, 0, 0)
ref_plane "to_frame_cap2_YZ" through (0, 0, -300) normal (1, 0, 0) x (0, -1, 0)
ref_plane "to_frame_cap2_ZX" through (0, 0, -300) normal (0, -1, 0) x (0, 0, -1)
body "Solid1"
